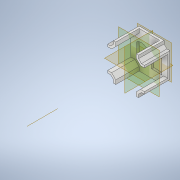
# Autodesk Inventor part: 20_Cube_Insert_Template_fullcube_v3
Saved by Autodesk Inventor 2022 (Build 260153000, 153)
## iProperties
Created: 2021-04-25
Part Number: 20_Cube_Insert_Template_fullcube_v3
Material: Generic
Document SubType Name: Modeling
Designer: diederichbenedict
Density: 1 g/cm^3
Appearance: Smooth - White
Author: diederichbenedict
Autodesk Inventor part; units mm, degrees
ref_plane "YZ Plane" through (0, 0, 0) normal (1, 0, 0) x (0, 1, 0)
ref_plane "XZ Plane" through (0, 0, 0) normal (0, 1, 0) x (-1, 0, 0)
ref_plane "Work Plane1" through (0, 0, -1) normal (0, 0, 1) x (1, 0, 0)
sketch "Sketch1" plane through (0, 0, -1) normal (0, 0, 1) x (1, 0, 0)
  arc A0 (24.85, 22.85) -> (22.85, 24.85) centre (22.85, 22.85) ccw construction
  line L0 (22.85, 24.85) -> (-16.97, 24.85) construction
  line L1 (-16.97, 24.85) -> (-16.97, 21.15) construction
  line L2 (-16.97, 21.15) -> (16.97, 21.15) construction
  line L3 (16.97, 16.97) -> (16.97, 21.15) construction
  line L4 (21.15, 16.97) -> (16.97, 16.97) construction
  line L5 (21.15, 16.97) -> (21.15, -16.97) construction
  line L6 (21.15, -16.97) -> (24.85, -16.97) construction
  line L7 (24.85, -16.97) -> (24.85, 22.85) construction
  line L8 (23.75, 23.25) -> (23.75, 18.15) construction
  arc A1 (23.25, 17.65) -> (23.75, 18.15) centre (23.25, 18.15) ccw construction
  line L9 (23.25, 17.65) -> (20.8937, 17.65) construction
  arc A2 (20.5239, 17.8134) -> (20.8937, 17.65) centre (20.8937, 18.15) ccw construction
  line L10 (20.5239, 17.8134) -> (17.7803, 20.8273) construction
  arc A3 (17.65, 21.1639) -> (17.7803, 20.8273) centre (18.15, 21.1639) ccw construction
  line L11 (17.65, 21.1639) -> (17.65, 23.25) construction
  arc A4 (18.15, 23.75) -> (17.65, 23.25) centre (18.15, 23.25) ccw construction
  line L12 (18.15, 23.75) -> (23.25, 23.75) construction
  arc A5 (23.75, 23.25) -> (23.25, 23.75) centre (23.25, 23.25) ccw construction
  arc A6 (-24.85, -22.85) -> (-22.85, -24.85) centre (-22.85, -22.85) ccw construction
  line L13 (-22.85, -24.85) -> (16.97, -24.85) construction
  line L14 (16.97, -24.85) -> (16.97, -21.15) construction
  line L15 (16.97, -21.15) -> (-16.97, -21.15) construction
  line L16 (-16.97, -16.97) -> (-16.97, -21.15) construction
  line L17 (-21.15, -16.97) -> (-16.97, -16.97) construction
  line L18 (-21.15, -16.97) -> (-21.15, 16.97) construction
  line L19 (-21.15, 16.97) -> (-24.85, 16.97) construction
  line L20 (-24.85, 16.97) -> (-24.85, -22.85) construction
  line L21 (-20.8273, -17.7803) -> (-17.8134, -20.5239) construction
  arc A7 (-17.65, -20.8937) -> (-17.8134, -20.5239) centre (-18.15, -20.8937) ccw construction
  line L22 (-17.65, -20.8937) -> (-17.65, -23.25) construction
  arc A8 (-18.15, -23.75) -> (-17.65, -23.25) centre (-18.15, -23.25) ccw construction
  line L23 (-18.15, -23.75) -> (-23.25, -23.75) construction
  arc A9 (-23.75, -23.25) -> (-23.25, -23.75) centre (-23.25, -23.25) ccw construction
  line L24 (-23.75, -23.25) -> (-23.75, -18.15) construction
  arc A10 (-23.25, -17.65) -> (-23.75, -18.15) centre (-23.25, -18.15) ccw construction
  line L25 (-23.25, -17.65) -> (-21.1639, -17.65) construction
  arc A11 (-20.8273, -17.7803) -> (-21.1639, -17.65) centre (-21.1639, -18.15) ccw construction
  arc A12 (-22.85, 24.85) -> (-24.85, 22.85) centre (-22.85, 22.85) ccw construction
  line L26 (-22.85, 24.85) -> (16.97, 24.85) construction
  line L27 (16.97, 24.85) -> (16.97, 21.15) construction
  line L28 (16.97, 21.15) -> (-16.97, 21.15) construction
  line L29 (-16.97, 16.97) -> (-16.97, 21.15) construction
  line L30 (-21.15, 16.97) -> (-16.97, 16.97) construction
  line L31 (-21.15, 16.97) -> (-21.15, -16.97) construction
  line L32 (-21.15, -16.97) -> (-24.85, -16.97) construction
  line L33 (-24.85, -16.97) -> (-24.85, 22.85) construction
  line L34 (-20.8273, 17.7803) -> (-17.8134, 20.5239) construction
  arc A13 (-17.8134, 20.5239) -> (-17.65, 20.8937) centre (-18.15, 20.8937) ccw construction
  line L35 (-17.65, 20.8937) -> (-17.65, 23.25) construction
  arc A14 (-17.65, 23.25) -> (-18.15, 23.75) centre (-18.15, 23.25) ccw construction
  line L36 (-18.15, 23.75) -> (-23.25, 23.75) construction
  arc A15 (-23.25, 23.75) -> (-23.75, 23.25) centre (-23.25, 23.25) ccw construction
  line L37 (-23.75, 23.25) -> (-23.75, 18.15) construction
  arc A16 (-23.75, 18.15) -> (-23.25, 17.65) centre (-23.25, 18.15) ccw construction
  line L38 (-23.25, 17.65) -> (-21.1639, 17.65) construction
  arc A17 (-21.1639, 17.65) -> (-20.8273, 17.7803) centre (-21.1639, 18.15) ccw construction
  arc A18 (22.85, -24.85) -> (24.85, -22.85) centre (22.85, -22.85) ccw construction
  line L39 (22.85, -24.85) -> (-16.97, -24.85) construction
  line L40 (-16.97, -24.85) -> (-16.97, -21.15) construction
  line L41 (-16.97, -21.15) -> (16.97, -21.15) construction
  line L42 (16.97, -16.97) -> (16.97, -21.15) construction
  line L43 (21.15, -16.97) -> (16.97, -16.97) construction
  line L44 (21.15, -16.97) -> (21.15, 16.97) construction
  line L45 (21.15, 16.97) -> (24.85, 16.97) construction
  line L46 (24.85, 16.97) -> (24.85, -22.85) construction
  line L47 (23.75, -23.25) -> (23.75, -18.15) construction
  arc A19 (23.75, -18.15) -> (23.25, -17.65) centre (23.25, -18.15) ccw construction
  line L48 (23.25, -17.65) -> (20.8937, -17.65) construction
  arc A20 (20.8937, -17.65) -> (20.5239, -17.8134) centre (20.8937, -18.15) ccw construction
  line L49 (20.5239, -17.8134) -> (17.7803, -20.8273) construction
  arc A21 (17.7803, -20.8273) -> (17.65, -21.1639) centre (18.15, -21.1639) ccw construction
  line L50 (17.65, -21.1639) -> (17.65, -23.25) construction
  arc A22 (17.65, -23.25) -> (18.15, -23.75) centre (18.15, -23.25) ccw construction
  line L51 (18.15, -23.75) -> (23.25, -23.75) construction
  arc A23 (23.25, -23.75) -> (23.75, -23.25) centre (23.25, -23.25) ccw construction
  line L52 (24.85, 16.87) -> (16.87, 16.87)
  line L53 (16.87, 16.87) -> (16.87, -16.87)
  line L54 (16.87, -16.87) -> (24.85, -16.87)
  line L55 (24.85, -16.87) -> (24.85, 16.87)
  line L56 (-16.87, 24.85) -> (16.87, 24.85)
  line L57 (16.87, 24.85) -> (16.87, 13.87)
  line L58 (16.87, 13.87) -> (-16.87, 13.87)
  line L59 (-16.87, 13.87) -> (-16.87, 24.85)
  line L60 (-16.87, 16.87) -> (-24.85, 16.87)
  line L61 (-24.85, 16.87) -> (-24.85, -16.87)
  line L62 (-24.85, -16.87) -> (-16.87, -16.87)
  line L63 (-16.87, -16.87) -> (-16.87, 16.87)
  line L64 (-16.87, -24.85) -> (16.87, -24.85)
  line L65 (16.87, -24.85) -> (16.87, -13.87)
  line L66 (16.87, -13.87) -> (-16.87, -13.87)
  line L67 (-16.87, -13.87) -> (-16.87, -24.85)
  arc A24 (12.6573, -5.8482) -> (12.7994, -6.05) centre (12.9383, -5.8013) ccw construction
  line L68 (12.7994, -6.05) -> (16.97, -6.05) construction
  line L69 (16.97, -6.05) -> (16.97, 6.05) construction
  line L70 (12.7994, 6.05) -> (16.97, 6.05) construction
  arc A25 (12.7994, 6.05) -> (12.6573, 5.8482) centre (12.9383, 5.8013) ccw construction
  arc A26 (12.2641, 5.5514) -> (12.6573, 5.8482) centre (11.7553, 6.6343) ccw construction
  arc A27 (12.2641, 5.5514) -> (12.1529, 5.425) centre (12.3846, 5.3332) ccw construction
  line L71 (12.1141, 4.928) -> (12.1529, 5.425) construction
  arc A28 (11.8955, 4.7) -> (12.1141, 4.928) centre (11.8656, 4.9475) ccw construction
  line L72 (11.4444, 4.7) -> (11.8955, 4.7) construction
  arc A29 (11.1961, 4.9275) -> (11.4444, 4.7) centre (11.4444, 4.9493) ccw construction
  line L73 (11.1642, 5.293) -> (11.1961, 4.9275) construction
  arc A30 (11.1642, 5.293) -> (11.0112, 5.5514) centre (10.9164, 5.3208) ccw construction
  arc A31 (10.4933, 5.8954) -> (11.0112, 5.5514) centre (11.4026, 6.7024) ccw construction
  arc A32 (10.4933, 5.8954) -> (10.27, 6.05) centre (10.2627, 5.8008) ccw construction
  line L74 (9.67, 6.05) -> (10.27, 6.05) construction
  line L75 (9.17, 5.55) -> (9.67, 6.05) construction
  line L76 (9.17, 5.55) -> (9.17, -5.55) construction
  line L77 (9.17, -5.55) -> (9.67, -6.05) construction
  line L78 (9.67, -6.05) -> (10.27, -6.05) construction
  arc A33 (10.27, -6.05) -> (10.4933, -5.8954) centre (10.2627, -5.8008) ccw construction
  arc A34 (11.0112, -5.5514) -> (10.4933, -5.8954) centre (11.4026, -6.7024) ccw construction
  arc A35 (11.0112, -5.5514) -> (11.1642, -5.293) centre (10.9164, -5.3208) ccw construction
  line L79 (11.1642, -5.293) -> (11.1961, -4.9275) construction
  arc A36 (11.4444, -4.7) -> (11.1961, -4.9275) centre (11.4444, -4.9493) ccw construction
  line L80 (11.4444, -4.7) -> (11.8955, -4.7) construction
  arc A37 (12.1141, -4.928) -> (11.8955, -4.7) centre (11.8656, -4.9475) ccw construction
  line L81 (12.1141, -4.928) -> (12.1529, -5.425) construction
  arc A38 (12.1529, -5.425) -> (12.2641, -5.5514) centre (12.3846, -5.3332) ccw construction
  arc A39 (12.6573, -5.8482) -> (12.2641, -5.5514) centre (11.7553, -6.6343) ccw construction
  circle A40 centre (-22.53, 11.5) radius 1.025 construction
  circle A41 centre (-22.53, -11.5) radius 1.025 construction
  line L82 (-11.03, -14.1) -> (-11.03, -12.75) construction
  arc A42 (-11.03, 12.75) -> (-11.03, -12.75) centre (-11.03, 0) ccw construction
  line L83 (-11.03, 12.75) -> (-11.03, 14.1) construction
  line L84 (-11.03, 14.1) -> (-22.53, 14.1) construction
  arc A43 (-22.53, 14.1) -> (-25.13, 11.5) centre (-22.53, 11.5) ccw construction
  line L85 (-25.13, 11.5) -> (-25.13, -11.5) construction
  arc A44 (-25.13, -11.5) -> (-22.53, -14.1) centre (-22.53, -11.5) ccw construction
  line L86 (-22.53, -14.1) -> (-11.03, -14.1) construction
  circle A45 centre (-11.03, 0) radius 12.75 construction
  circle A46 centre (0.47, 11.5) radius 1.025 construction
  circle A47 centre (0.47, -11.5) radius 1.025 construction
  circle A48 centre (-22.53, -11.5) radius 1.025 construction
  circle A49 centre (-22.53, 11.5) radius 1.025 construction
  line L87 (-22.53, -14.1) -> (0.47, -14.1) construction
  arc A50 (-25.13, -11.5) -> (-22.53, -14.1) centre (-22.53, -11.5) ccw construction
  line L88 (-25.13, 11.5) -> (-25.13, -11.5) construction
  arc A51 (-22.53, 14.1) -> (-25.13, 11.5) centre (-22.53, 11.5) ccw construction
  line L89 (0.47, 14.1) -> (-22.53, 14.1) construction
  arc A52 (3.07, 11.5) -> (0.47, 14.1) centre (0.47, 11.5) ccw construction
  line L90 (3.07, -11.5) -> (3.07, 11.5) construction
  arc A53 (0.47, -14.1) -> (3.07, -11.5) centre (0.47, -11.5) ccw construction
  line L91 (-16.87, 13.87) -> (3.07, 13.87)
  line L92 (3.07, 13.87) -> (3.07, -13.87)
  line L93 (3.07, -13.87) -> (-16.87, -13.87)
  line L94 (-16.87, -13.87) -> (-16.87, 13.87)
  circle A54 centre (-11.03, 0) radius 2.75 construction
  arc A55 (-16.87, -7.9971) -> (-16.87, 7.9971) centre (-11.03, 0) ccw
  line L95 (-16.87, 7.9971) -> (-16.87, -7.9971)
  point P0 (0, 0)
  dimension "d1" = 0.1
  dimension "d2" = 0.1
  dimension "d3" = 0.1
  dimension "d4" = 0.1
  dimension "d5" = 0.1
  dimension "d6" = 3
  dimension "d7" = 3
  constraints: 42 end point, 11 point on line, 10 parallel, 5 horizontal, 5 perpendicular, 2 point on circle, 1 centre point, 1 coincident, 1 collinear
  measures "d1" distance between parallel lines of L30 L60
  measures "d2" distance between parallel lines of L1 L59
  measures "d3" distance between parallel lines of L27 L57
  measures "d4" distance between parallel lines of L43 L54
  measures "d5" distance between parallel lines of L16 L67
  measures "d6" distance between parallel lines of L60 L58
  measures "d7" distance between parallel lines of L62 L66
extrude "Extrusion1" add sketch "Sketch1" along normal blind 3 contours L55 L54 L53 L52 | L53 L58 L59 L56 L57 | L65 L64 L67 L63 L66 L53 | L92 L66 L63 A55 L58 | L63 L62 L61 L60 L59
chamfer "Chamfer1" distance 3.9 angle 45 4 edges at (16.87, -16.87, 0.5) (-16.87, -16.87, 0.5) (-16.87, 16.87, 0.5) (16.87, 16.87, 0.5)
sketch "Sketch2" plane through (0, 0, 2) normal (0, 0, 1) x (1, 0, 0)
  line L0 (3.07, 13.87) -> (16.87, 13.87) projected
  line L1 (16.87, 13.87) -> (16.87, -13.87) projected
  line L2 (16.87, -13.87) -> (3.07, -13.87) projected
  line L3 (-16.87, -20.77) -> (-16.87, -24.85) projected
  line L4 (-16.87, -24.85) -> (16.87, -24.85) projected
  line L5 (16.87, -24.85) -> (16.87, -20.77) projected
  line L6 (20.77, -16.87) -> (16.87, -20.77) projected
  line L7 (20.77, -16.87) -> (24.85, -16.87) projected
  line L8 (24.85, -16.87) -> (24.85, 16.87) projected
  line L9 (24.85, 16.87) -> (20.77, 16.87) projected
  line L10 (16.87, 20.77) -> (20.77, 16.87) projected
  line L11 (16.87, 20.77) -> (16.87, 24.85) projected
  line L12 (16.87, 24.85) -> (-16.87, 24.85) projected
  line L13 (-16.87, 24.85) -> (-16.87, 20.77) projected
  line L14 (-20.77, 16.87) -> (-16.87, 20.77) projected
  line L15 (-20.77, 16.87) -> (-24.85, 16.87) projected
  line L16 (-24.85, 16.87) -> (-24.85, -16.87) projected
  line L17 (-24.85, -16.87) -> (-20.77, -16.87) projected
  line L18 (-16.87, -20.77) -> (-20.77, -16.87) projected
  line L19 (13.8689, -19.5269) -> (13.8689, -21.8489)
  line L20 (-13.8689, -21.8489) -> (-13.8689, -19.5269)
  line L21 (-13.8689, -19.5269) -> (-19.5269, -13.8689)
  line L22 (-19.5269, -13.8689) -> (-21.8489, -13.8689)
  line L23 (-21.8489, 13.8689) -> (-19.5269, 13.8689)
  line L24 (-19.5269, 13.8689) -> (-13.8689, 19.5269)
  line L25 (-13.8689, 19.5269) -> (-13.8689, 21.8489)
  line L26 (13.8689, 21.8489) -> (13.8689, 19.5269)
  line L27 (13.8689, 19.5269) -> (19.5269, 13.8689)
  line L28 (19.5269, 13.8689) -> (21.8489, 13.8689)
  line L29 (21.8489, -13.8689) -> (19.5269, -13.8689)
  line L30 (19.5269, -13.8689) -> (13.8689, -19.5269)
  line L31 (13.8689, -21.8489) -> (13.8689, -24.85)
  line L32 (16.87, -24.85) -> (-16.87, -24.85) projected
  line L33 (21.8489, -13.8689) -> (24.85, -13.8689)
  line L34 (24.85, -16.87) -> (24.85, 16.87) projected
  line L35 (21.8489, 13.8689) -> (24.85, 13.8689)
  line L36 (13.8689, 21.8489) -> (13.8689, 24.85)
  line L37 (-13.8689, 21.8489) -> (-13.8689, 24.85)
  line L38 (-21.8489, 13.8689) -> (-24.85, 13.8689)
  line L39 (-21.8489, -13.8689) -> (-24.85, -13.8689)
  line L40 (-13.8689, -21.8489) -> (-13.8689, -24.85)
  line L41 (13.8689, -21.8489) -> (11.5469, -21.8489)
  line L42 (-11.5469, -21.8489) -> (-13.8689, -21.8489)
  line L43 (21.8489, 13.8689) -> (21.8489, 11.5469)
  line L44 (21.8489, -11.5469) -> (21.8489, -13.8689)
  line L45 (-21.8489, -13.8689) -> (-21.8489, -11.5469)
  line L46 (-21.8489, 11.5469) -> (-21.8489, 13.8689)
  line L47 (-13.8689, 21.8489) -> (-11.5469, 21.8489)
  line L48 (11.5469, 21.8489) -> (13.8689, 21.8489)
  line L49 (3.07, -13.87) -> (3.07, 13.87) projected
  point P0 (0, 0)
  dimension "d13" = 3.0011
  constraints: 56 end point, 20 point on line, 3 perpendicular, 1 parallel, 7 other
  measures "d13" distance between parallel lines of L5 L19
ref_plane "Work Plane2" through (-16.97, -24.85, 34.1) normal (0, 0, -1) x (0, 1, 0)
extrude "Extrusion2" add sketch "Sketch2" along normal blind 31.5 contours L31 L19 L30 L29 L33 L8 L7 L6 L5 L4
pattern_circular "Circular Pattern1" count 4 over 360 about axis through (0, 0, 146.63) along (0, 0, -1) of "Extrusion2"
ref_plane "Work Plane9" through (-16.87, 0, -1) normal (0, 1, 0) x (1, 0, 0)
ref_plane "Work Plane10" through (0, -16.87, -1) normal (-1, 0, 0) x (0, 0, 1)
ref_plane "Work Plane11" through (0, 0, 16.25) normal (0, 0, -1) x (-1, 0, 0)
equation "\"d2\" = d1"
equation "\"d3\" = d1"
equation "\"d4\" = d1"
equation "\"d5\" = d1"
body "Solid1"
